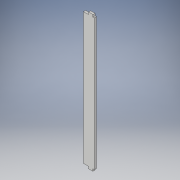
# Autodesk Inventor part: 3 binnen dunne cover plaat
Saved by Autodesk Inventor 2019 (Build 230136000, 136)
## iProperties
Created: 2021-01-22
Part Number: 3 binnen dunne cover plaat
Material: Generic
Document SubType Name: Sheet Metal
Designer: Stefan
Density: 1 g/cm^3
Sheet Metal Rule: Default_mm
Appearance: Default
Author: Stefan
Autodesk Inventor part; units mm, degrees
ref_plane "YZ Plane" through (0, 0, 0) normal (1, 0, 0) x (0, 1, 0)
ref_plane "XZ Plane" through (0, 0, 0) normal (0, 1, 0) x (-1, 0, 0)
ref_plane "XY Plane" through (0, 0, 0) normal (0, 0, 1) x (1, 0, 0)
sketch "Sketch1" plane through (0, 0, 0) normal (0, 0, 1) x (1, 0, 0)
  line L0 (5, -90.5) -> (5, 90.5)
  line L1 (-5, -90.5) -> (5, 90.5) construction
  line L2 (5, -90.5) -> (-5, 90.5) construction
  line L3 (3, 90.5) -> (3, 93.5)
  line L4 (3, 93.5) -> (-3, 93.5)
  line L5 (-3, 93.5) -> (-3, 90.5)
  line L6 (5, 90.5) -> (3, 90.5)
  line L7 (-3, 90.5) -> (-5, 90.5)
  line L8 (3, -90.5) -> (3, -93.5)
  line L9 (3, -93.5) -> (-3, -93.5)
  line L10 (-3, -93.5) -> (-3, -90.5)
  line L11 (-5, -90.5) -> (-3, -90.5)
  line L12 (3, -90.5) -> (5, -90.5)
  line L13 (-5, -90.5) -> (-10, -90.5)
  line L14 (-10, -90.5) -> (-10, 90.5)
  line L15 (-10, 90.5) -> (-5, 90.5)
  point P0 (0, 0)
  dimension "d0" = 10
  dimension "d1" = 181
  dimension "d2" = 6
  dimension "d3" = 3
  dimension "d5" = 6
  dimension "d6" = 3
  dimension "d8" = 3.162
  dimension "d9" = 3.162
  dimension "d12" = 5
  dimension "d13" = 90
  dimension "d14" = 2
  dimension "d15" = 15
  dimension "d16" = 3
  constraints: 32 end point, 9 parallel, 4 perpendicular, 3 horizontal, 2 midpoint
  measures "d0" distance of L2.end L0.end
  measures "d1" distance of L0.end L0.start
  measures "d2" distance of L4.end L3.end
  measures "d3" distance of L3.end L3.start
  measures "d5" distance of L8.end L9.end
  measures "d6" distance of L8.start L8.end
  measures "d8" angle of L2 L0
  measures "d9" angle of L1 L0
  measures "d12" distance of L1.start L13.end
  measures "d13" angle of L6 L8
  measures "d14" distance between parallel lines of L3 L0
  measures "d15" distance between parallel lines of L14 L0
  measures "d16" distance from line of point (0, 0) L8
extrude "Extrusion1" add sketch "Sketch1" along normal blind 3
equation "\"BendRadius\" = Thickness"
equation "\"BendReliefWidth\" = Thickness"
equation "\"BendReliefDepth\" = 0.5 * Thickness"
equation "\"CornerReliefSize\" = 4 * Thickness"
equation "\"MinimumRemnant\" = 2 * Thickness"
equation "\"TransitionRadius\" = BendRadius"
equation "\"JacobiRadiusSize\" = BendRadius"
equation "\"GapSize\" = Thickness"
equation "\"Thickness\" = 0.5"
body "Solid1"
